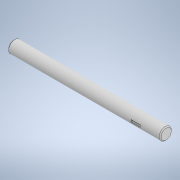
# Autodesk Inventor part: Mainpulo
Saved by Autodesk Inventor 2021 (Build 250183000, 183)
## iProperties
Created: 2022-02-22
Part Number: Mainpulo
Material: Genérico
Document SubType Name: Modeling
Designer: aluno
Density: 1 g/cm^3
Appearance: Padrão
Author: aluno
Autodesk Inventor part; units mm, degrees
ref_plane "YZ Plane" through (0, 0, 0) normal (1, 0, 0) x (0, 1, 0)
ref_plane "XZ Plane" through (0, 0, 0) normal (0, 1, 0) x (-1, 0, 0)
ref_plane "XY Plane" through (0, 0, 0) normal (0, 0, 1) x (1, 0, 0)
sketch "Esboço1" plane through (0, 0, 0) normal (0, 0, 1) x (1, 0, 0)
  line L0 (0, 0) -> (75, 0)
  line L1 (75, 0) -> (75, 3)
  line L2 (75, 3) -> (0, 3)
  line L3 (0, 3) -> (0, 0)
  dimension "d0" = 75
  dimension "d1" = 3
  constraints: 8 end point, 2 parallel, 1 horizontal, 1 perpendicular
  measures "d0" distance of L2.end L1.end
  measures "d1" distance of L1.end L0.end
revolve "Revolução1" add sketch "Esboço1" angle 360 about axis through (0, 0, 0) along (1, 0, 0)
sketch "Esboço2" plane through (0, 0, 0) normal (0, 1, 0) x (-1, 0, 0)
  point P0 (0, 0)
chamfer "Chanfro1" distance 0.5 angle 45 2 edges at (0, -3, 0) (75, -3, 0)
sketch "Esboço3" plane through (0, 0, 0) normal (0, 1, 0) x (-1, 0, 0)
  circle A0 centre (-12, -2) radius 2.5
  line L0 (0, 2.5) -> (0, -2.5) projected
  line L1 (-75, 2.5) -> (-74.5, 3) projected
  line L2 (-74.5, 3) -> (-0.5, 3) projected
  line L3 (-0.5, 3) -> (0, 2.5) projected
  line L4 (0, 2.5) -> (0, -2.5) projected
  line L5 (0, -2.5) -> (-0.5, -3) projected
  line L6 (-0.5, -3) -> (-74.5, -3) projected
  line L7 (-74.5, -3) -> (-75, -2.5) projected
  line L8 (-75, -2.5) -> (-75, 2.5) projected
  circle A1 centre (-63, 2) radius 2.5
  line L9 (-0.5, -3) -> (-74.5, -3) projected
  line L10 (-9.5, -2) -> (-14.5, -2)
  line L11 (-14.5, -2) -> (-14.5, -3)
  line L12 (-14.5, -3) -> (-9.5, -3)
  line L13 (-9.5, -3) -> (-9.5, -2)
  line L14 (-60.5, 2) -> (-65.5, 2)
  line L15 (-65.5, 2) -> (-65.5, 3)
  line L16 (-65.5, 3) -> (-60.5, 3)
  line L17 (-60.5, 3) -> (-60.5, 2)
  point P0 (0, 0)
  point P1 (-9.7087, -3)
  point P2 (-14.2913, -3)
  dimension "d6" = 5
  dimension "d9" = 5
  dimension "d10" = 12
  dimension "d11" = 1.5
  dimension "d12" = 12
  dimension "d13" = 1.5
  constraints: 16 end point, 4 parallel, 2 horizontal, 2 perpendicular, 2 point on line, 1 horizontal alignment, 5 other
  measures "d10" distance from line of L8 point (-63, 2)
  measures "d12" distance from line of L0 point (-12, -2)
extrude "Extrusão1" cut sketch "Esboço3" against normal mid plane 1 contours L10 A0 | A0 L6 L10 | A0 L6 | A1 L14 L2 | L2 A1 | A1 L14
